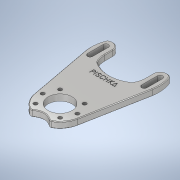
# Autodesk Inventor part: Motor Holder v3
Saved by Autodesk Inventor 2020.1 (Build 241239000, 239)
## iProperties
Created: 2019-03-01
Part Number: Motor Holder v3
Material: Aluminum 6061-AHC
Document SubType Name: Modeling
Designer: Petar
Density: 2.7 g/cm^3
Appearance: Aluminum - Dark
Mass: 26.5004 g
Surface Area: 70.5339 cm^2
Volume: 9.81495 cm^3
Author: Petar
Autodesk Inventor part; units mm, degrees
ref_plane "YZ Plane" through (0, 0, 0) normal (1, 0, 0) x (0, 1, 0)
ref_plane "XZ Plane" through (0, 0, 0) normal (0, 1, 0) x (-1, 0, 0)
ref_plane "XY Plane" through (0, 0, 0) normal (0, 0, 1) x (1, 0, 0)
sketch "Sketch1" plane through (0, 0, 0) normal (0, 1, 0) x (-1, 0, 0)
  line L0 (0, 0) -> (0, 51.5) construction
  circle A0 centre (0, 51.5) radius 9.5
  line L1 (16, -6.25) -> (16, 0)
  line L2 (21.5, 19.91967) -> (21.5, -14.08033) construction
  line L3 (-21.5, 18) -> (-21.5, -16) construction
  circle A1 centre (21.5, 3.5) radius 1.75 construction
  circle A2 centre (21.5, -3.5) radius 1.75 construction
  circle A3 centre (-21.5, 3.5) radius 1.75 construction
  circle A4 centre (-21.5, -3.5) radius 1.75 construction
  line L4 (-16, -6.25) -> (-16, 0)
  line L5 (21.5, 6.25) -> (21.5, -6.25) construction
  line L6 (19.45, 6.25) -> (19.45, -6.25)
  line L7 (23.55, -6.25) -> (23.55, 6.25)
  arc A5 (23.55, 6.25) -> (19.45, 6.25) centre (21.5, 6.25) ccw
  arc A6 (19.45, -6.25) -> (23.55, -6.25) centre (21.5, -6.25) ccw
  line L8 (-19.45, 6.25) -> (-19.45, -6.25)
  line L9 (-23.55, -6.25) -> (-23.55, 6.25)
  arc A7 (-19.45, 6.25) -> (-23.55, 6.25) centre (-21.5, 6.25) ccw
  arc A8 (-23.55, -6.25) -> (-19.45, -6.25) centre (-21.5, -6.25) ccw
  arc A9 (14.544724, 41.768556) -> (17.199681, 54.728155) centre (0, 51.5) ccw construction
  arc A10 (16, -6.25) -> (24.816002, -10.637953) centre (21.5, -6.25) ccw
  arc A11 (-24.816002, -10.637953) -> (-16, -6.25) centre (-21.5, -6.25) ccw
  line L10 (17.199681, 54.728155) -> (26.53665, 4.980583)
  line L11 (-17.199681, 54.728155) -> (-26.53665, 4.980583)
  circle A12 centre (0, 51.5) radius 13.75 construction
  circle A13 centre (9.722718, 61.222718) radius 1.5
  circle A14 centre (9.722718, 41.777282) radius 1.5
  line L12 (0, 51.5) -> (9.722718, 61.222718) construction
  line L13 (9.722718, 41.777282) -> (0, 51.5) construction
  circle A15 centre (-9.722718, 61.222718) radius 1.5
  circle A16 centre (-9.722718, 41.777282) radius 1.5
  circle A17 centre (13.75, 51.5) radius 1.5
  line L14 (13.75, 51.5) -> (0, 51.5) construction
  circle A18 centre (-13.75, 51.5) radius 1.5
  circle A19 centre (0, 22.942114) radius 1.5 construction
  line L15 (14.544724, 41.768556) -> (18.735106, 19.442114) construction
  arc A20 (17.199681, 54.728155) -> (-17.199681, 54.728155) centre (0, 51.5) ccw
  arc A21 (-17.199681, 54.728155) -> (-14.544724, 41.768556) centre (0, 51.5) ccw construction
  line L16 (-14.544724, 41.768556) -> (-18.735106, 19.442114) construction
  line L17 (7.5, 67.311388) -> (0, 61) construction
  line L18 (0, 61) -> (-7.5, 67.311388) construction
  spline S0 degree 2 poles (7.5, 67.311388) (0, 61) (-7.5, 67.311388) knots 1 1 1 2 2 2
  line L19 (7.5, 67.311388) -> (-7.5, 67.311388) construction
  line L20 (18.735106, 19.442114) -> (-18.735106, 19.442114) construction
  line L21 (18.735106, 19.442114) -> (11.806239, 33.884362) construction
  line L22 (14.544724, 41.768556) -> (12.108743, 38.127711) construction
  arc A22 (12.108743, 38.127711) -> (11.806239, 33.884362) centre (15.676028, 35.740946) ccw construction
  line L23 (-18.735106, 19.442114) -> (-11.806239, 33.884362) construction
  line L24 (-14.544724, 41.768556) -> (-12.108743, 38.127711) construction
  arc A23 (-11.806239, 33.884362) -> (-12.108743, 38.127711) centre (-15.676028, 35.740946) ccw construction
  line L25 (14.298579, 19.442114) -> (8.163141, 32.230571) construction
  line L26 (14.298579, 19.442114) -> (7.49461, 25.938983) construction
  line L27 (8.163141, 32.230571) -> (6.995239, 30.485011) construction
  arc A24 (6.995239, 30.485011) -> (7.49461, 25.938983) centre (9.94862, 28.508992) ccw construction
  line L28 (-14.298579, 19.442114) -> (-8.163141, 32.230571) construction
  line L29 (-14.298579, 19.442114) -> (-7.49461, 25.938983) construction
  line L30 (-8.163141, 32.230571) -> (-6.995239, 30.485011) construction
  arc A25 (-7.49461, 25.938983) -> (-6.995239, 30.485011) centre (-9.94862, 28.508992) ccw construction
  arc A26 (24.816002, -10.637953) -> (27, 0) centre (0, 0) ccw
  arc A27 (-24.816002, -10.637953) -> (24.816002, -10.637953) centre (0, 0) ccw construction
  arc A28 (-10.270866, 24.970168) -> (-26.53665, 4.980583) centre (0, 0) ccw construction
  line L31 (21.5, -11.75) -> (-21.5, -11.75) construction
  line L32 (-21.213203, 69) -> (25, 69) construction
  line L33 (0, 61) -> (0, 61) construction
  arc A29 (13.760985, 8.163043) -> (-13.760985, 8.163043) centre (0, -11.5) ccw
  line L34 (13.760985, 8.163043) -> (-13.760985, 8.163043) construction
  arc A30 (16, 0) -> (13.760985, 8.163043) centre (0, 0) ccw
  arc A31 (-13.760985, 8.163043) -> (-16, 0) centre (0, 0) ccw
  arc A32 (27, 0) -> (26.53665, 4.980583) centre (0, 0) ccw
  arc A33 (-27, 0) -> (-24.816002, -10.637953) centre (0, 0) ccw
  arc A34 (-26.53665, 4.980583) -> (-27, 0) centre (0, 0) ccw
  arc A35 (26.53665, 4.980583) -> (-12.029232, 24.172248) centre (0, 0) ccw construction
  line L35 (16, 0) -> (-16, 0) construction
  point P0 (21.5, 0)
  point P1 (0, 12.5)
  dimension "d1" = 19
  dimension "d0" = 51.5
  dimension "d3" = 3.5
  dimension "d4" = 3.5
  dimension "d5" = 7
  dimension "d9" = 3.5
  dimension "d11" = 32
  dimension "d15" = 4.1
  dimension "d24" = 3
  dimension "d25" = 3
  dimension "d27" = 45
  dimension "d29" = 3
  dimension "d30" = 3
  dimension "d50" = 15
  dimension "d53" = 27
  dimension "d75" = 80.75
  dimension "d76" = 8
  dimension "d78" = 0
  dimension "d81" = 6.25
  dimension "d82" = 12.5
  dimension "d85" = 5
  dimension "d86" = 4
  dimension "d98" = 15
  dimension "d99" = 24
  dimension "d101" = 43
  dimension "d104" = 2
  dimension "d105" = 27.5
  constraints: 70 end point, 58 point on circle, 35 centre point, 26 symmetric about line, 19 tangent, 13 point on line, 7 coincident, 5 horizontal, 5 vertical, 3 parallel, 2 perpendicular, 1 collinear, 1 midpoint, 1 vertical alignment, 16 other
  measures "d0" distance of L0.start L0.end
  measures "d3" diameter of A1
  measures "d4" diameter of A2
  measures "d5" distance of A2.centre A1.centre
  measures "d9" vertical distance of L0.start A1.centre
  measures "d11" distance between parallel lines of L4 L1
  measures "d15" distance between parallel lines of L6 L7
  measures "d24" diameter of A13
  measures "d25" diameter of A14
  measures "d27" angle of L0 L13
  measures "d29" diameter of A17
  measures "d30" diameter of A19
  measures "d50" distance of L17.start L18.end
  measures "d53" radius of A26
  measures "d75" distance between parallel lines of L31 L32
  measures "d78" distance of L33.start L33.end
  measures "d81" vertical distance of L5.start point (0, 12.5)
  measures "d82" distance of L5.end L5.start
  measures "d85" distance between parallel lines of L10 L15
  measures "d86" distance between parallel lines of L21 L25
  measures "d98" angle of L15 L21
  measures "d99" radius of A29
  measures "d101" distance of A4.centre A2.centre
  measures "d104" distance edge to line of A19 L20
  measures "d105" diameter of A12
extrude "Extrusion3" add sketch "Sketch1" along normal blind 5 contours L1 A30 A29 A31 L4 A11 A33 A34 L11 A20 S0 L10 A32 A26 A10
thread "Thread1" size "M3x0.5" class "6H" standard "ANSI Metric M Profile" full length
thread "Thread2" size "M3x0.5" class "6H" standard "ANSI Metric M Profile" full length
thread "Thread4" size "M3x0.5" class "6H" standard "ANSI Metric M Profile" full length
thread "Thread5" size "M3x0.5" class "6H" standard "ANSI Metric M Profile" full length
thread "Thread6" size "M3x0.5" class "6H" standard "ANSI Metric M Profile" full length
thread "Thread7" size "M3x0.5" class "6H" standard "ANSI Metric M Profile" full length
sketch "Sketch3" plane through (0, 5, 0) normal (0, 1, 0) x (1, 0, 0)
  line L0 (0, 0) -> (0, -51.5) construction
  circle A0 centre (0, -51.5) radius 9.5 construction
  arc A1 (-24.816002, 10.637953) -> (-26.53665, -4.980583) centre (0, 0) ccw construction
  line L1 (-7.003029, -18.212174) -> (-6.698457, -18.212174)
  line L2 (-7.003029, -14.734984) -> (-7.003029, -18.212174)
  line L3 (-6.698457, -18.212174) -> (-6.698457, -14.734984)
  spline S0 degree 3 poles (-5.654031, -15.648698) (-5.637534, -15.935503) (-5.515705, -16.141088) (-5.260627, -16.308603) knots 0 0 0 0 1 1 1 1
  spline S1 degree 3 poles (-5.04362, -16.066214) (-5.301236, -15.889817) (-5.388801, -15.600474) (-5.275855, -15.29971) knots 0 0 0 0 1 1 1 1
  spline S2 degree 3 poles (-5.275855, -15.29971) (-5.217479, -15.142348) (-5.041082, -15.007829) (-4.826613, -14.955798) knots 0 0 0 0 1 1 1 1
  spline S3 degree 3 poles (-4.858339, -14.684222) (-5.372303, -14.767979) (-5.68322, -15.143617) (-5.654031, -15.648698) knots 0 0 0 0 1 1 1 1
  spline S4 degree 3 poles (-4.744124, -14.665186) (-4.754277, -14.667724) (-4.806308, -14.676608) (-4.858339, -14.684222) knots 0 0 0 0 1 1 1 1
  line L4 (-6.698457, -14.734984) -> (-7.003029, -14.734984)
  line L5 (-9.769552, -16.702007) -> (-9.448483, -16.702007)
  spline S5 degree 3 poles (-9.448483, -16.702007) (-8.949748, -16.702007) (-8.673095, -16.669012) (-8.429438, -16.581448) knots 0 0 0 0 1 1 1 1
  line L6 (-10.074124, -14.732446) -> (-10.074124, -18.212174)
  line L7 (-9.769552, -18.212174) -> (-9.769552, -16.702007)
  line L8 (-10.074124, -18.212174) -> (-9.769552, -18.212174)
  spline S6 degree 3 poles (-7.845676, -15.941848) (-7.816488, -15.794638) (-7.826641, -15.519255) (-7.865981, -15.382198) knots 0 0 0 0 1 1 1 1
  spline S7 degree 3 poles (-8.429438, -16.581448) (-8.108369, -16.467233) (-7.906591, -16.246419) (-7.845676, -15.941848) knots 0 0 0 0 1 1 1 1
  spline S8 degree 3 poles (-7.865981, -15.382198) (-7.964967, -15.038286) (-8.199741, -14.854274) (-8.643907, -14.771786) knots 0 0 0 0 1 1 1 1
  spline S9 degree 3 poles (-8.161669, -15.648698) (-8.142633, -15.960884) (-8.256848, -16.186774) (-8.491621, -16.300988) knots 0 0 0 0 1 1 1 1
  spline S10 degree 3 poles (-8.623602, -15.062398) (-8.317762, -15.146155) (-8.183243, -15.318746) (-8.161669, -15.648698) knots 0 0 0 0 1 1 1 1
  spline S11 degree 3 poles (-8.491621, -16.300988) (-8.678171, -16.393629) (-8.81269, -16.410126) (-9.365995, -16.410126) knots 0 0 0 0 1 1 1 1
  line L9 (-9.365995, -16.410126) -> (-9.769552, -16.410126)
  line L10 (-9.769552, -16.410126) -> (-9.769552, -15.024327)
  spline S12 degree 3 poles (-4.528386, -16.300988) (-4.630505, -16.264595) (-4.739368, -16.222518) (-4.904133, -16.14744) (-4.983604, -16.107764) (-5.04362, -16.066214) knots -1.50825171 -1.50825171 -1.50825171 -1.50825171 -0.60874864 -0.60874864 0 0 0 0
  spline S13 degree 3 poles (-5.260627, -16.308603) (-5.126108, -16.397436) (-4.959863, -16.469772) (-4.598184, -16.595407) knots 0 0 0 0 1 1 1 1
  line L11 (-5.407836, -17.31115) -> (-5.735251, -17.31115)
  line L12 (-5.735251, -17.31115) -> (-5.726367, -17.370795)
  line L13 (-5.387532, -17.410136) -> (-5.407836, -17.31115)
  spline S14 degree 3 poles (-4.826613, -14.955798) (-4.706053, -14.925341) (-4.420517, -14.92661) (-4.280922, -14.955798) knots 0 0 0 0 1 1 1 1
  spline S15 degree 3 poles (-4.228891, -14.689298) (-4.321532, -14.671531) (-4.69717, -14.653765) (-4.744124, -14.665186) knots 0 0 0 0 1 1 1 1
  line L14 (-3.801222, -15.405041) -> (-3.785994, -15.483722)
  spline S16 degree 3 poles (-4.280922, -14.955798) (-4.010615, -15.014174) (-3.846908, -15.168998) (-3.801222, -15.405041) knots 0 0 0 0 1 1 1 1
  line L15 (-3.785994, -15.483722) -> (-3.473808, -15.483722)
  line L16 (-3.473808, -15.483722) -> (-3.482691, -15.435498)
  spline S17 degree 3 poles (-3.482691, -15.435498) (-3.523301, -15.198186) (-3.581677, -15.070012) (-3.708582, -14.943108) knots 0 0 0 0 1 1 1 1
  spline S18 degree 3 poles (-3.708582, -14.943108) (-3.845639, -14.807319) (-3.99031, -14.736253) (-4.228891, -14.689298) knots 0 0 0 0 1 1 1 1
  spline S19 degree 3 poles (-1.434449, -14.677877) (-1.881154, -14.750212) (-2.21872, -15.00656) (-2.428113, -15.430422) knots 0 0 0 0 1 1 1 1
  spline S20 degree 3 poles (-2.320244, -16.473579) (-2.320244, -15.682962) (-2.014404, -15.137272) (-1.487749, -14.986255) knots 0 0 0 0 1 1 1 1
  spline S21 degree 3 poles (-1.487749, -14.986255) (-1.402723, -14.962143) (-1.357037, -14.957067) (-1.190792, -14.957067) knots 0 0 0 0 1 1 1 1
  spline S22 degree 3 poles (-1.190792, -14.957067) (-1.01947, -14.957067) (-0.981399, -14.960874) (-0.898911, -14.986255) knots 0 0 0 0 1 1 1 1
  spline S23 degree 3 poles (-0.853225, -14.695643) (-0.991551, -14.661379) (-1.283432, -14.652496) (-1.434449, -14.677877) knots 0 0 0 0 1 1 1 1
  line L17 (-0.386216, -15.511641) -> (-0.378601, -15.547174)
  spline S24 degree 3 poles (-0.898911, -14.986255) (-0.612106, -15.077627) (-0.444592, -15.248948) (-0.386216, -15.511641) knots 0 0 0 0 1 1 1 1
  spline S25 degree 3 poles (-0.188244, -15.123312) (-0.32657, -14.91265) (-0.546116, -14.770517) (-0.853225, -14.695643) knots 0 0 0 0 1 1 1 1
  spline S26 degree 3 poles (-0.053725, -15.481184) (-0.068954, -15.370776) (-0.126061, -15.218491) (-0.188244, -15.123312) knots 0 0 0 0 1 1 1 1
  line L18 (-0.378601, -15.547174) -> (-0.044842, -15.547174)
  line L19 (-0.044842, -15.547174) -> (-0.053725, -15.481184)
  spline S27 degree 3 poles (-2.428113, -15.430422) (-2.64512, -15.869512) (-2.708572, -16.477386) (-2.594358, -17.033229) knots 0 0 0 0 1 1 1 1
  spline S28 degree 3 poles (-5.236515, -17.740088) (-5.299967, -17.661407) (-5.36342, -17.523081) (-5.387532, -17.410136) knots 0 0 0 0 1 1 1 1
  spline S29 degree 3 poles (-5.726367, -17.370795) (-5.699717, -17.553538) (-5.607077, -17.779428) (-5.505553, -17.905064) knots 0 0 0 0 1 1 1 1
  spline S30 degree 3 poles (-4.774582, -17.991359) (-4.867932, -17.973746) (-4.959865, -17.944336) (-5.117505, -17.858587) (-5.183697, -17.806111) (-5.236515, -17.740088) knots -1.49467749 -1.49467749 -1.49467749 -1.49467749 -0.70511356 -0.70511356 0 0 0 0
  spline S31 degree 3 poles (-5.505553, -17.905064) (-5.305043, -18.153797) (-4.956055, -18.288316) (-4.509351, -18.288316) knots 0 0 0 0 1 1 1 1
  spline S32 degree 3 poles (-9.245436, -15.029403) (-8.758121, -15.034479) (-8.716243, -15.037017) (-8.623602, -15.062398) knots 0 0 0 0 1 1 1 1
  spline S33 degree 3 poles (-8.643907, -14.771786) (-8.772081, -14.747674) (-8.846955, -14.743867) (-9.429447, -14.738791) knots 0 0 0 0 1 1 1 1
  line L20 (-9.429447, -14.738791) -> (-10.074124, -14.732446)
  line L21 (-9.769552, -15.024327) -> (-9.245436, -15.029403)
  spline S34 degree 3 poles (-0.731397, -17.893643) (-0.88622, -17.971055) (-0.975054, -17.99009) (-1.190792, -17.99009) knots 0 0 0 0 1 1 1 1
  spline S35 degree 3 poles (-0.386216, -17.434248) (-0.430632, -17.637295) (-0.558806, -17.806078) (-0.731397, -17.893643) knots 0 0 0 0 1 1 1 1
  spline S36 degree 3 poles (-1.108304, -18.28324) (-0.69967, -18.262936) (-0.36718, -18.09669) (-0.188244, -17.823845) knots 0 0 0 0 1 1 1 1
  line L22 (-0.378601, -17.399983) -> (-0.386216, -17.434248)
  line L23 (-0.046111, -17.399983) -> (-0.378601, -17.399983)
  line L24 (-0.054994, -17.465974) -> (-0.046111, -17.399983)
  spline S37 degree 3 poles (-0.188244, -17.823845) (-0.126061, -17.728667) (-0.070223, -17.57765) (-0.054994, -17.465974) knots 0 0 0 0 1 1 1 1
  line L25 (1.156946, -14.734984) -> (0.852375, -14.734984)
  line L26 (1.156946, -16.257841) -> (1.156946, -14.734984)
  line L27 (0.852375, -14.734984) -> (0.852375, -18.212174)
  line L28 (0.852375, -18.212174) -> (1.156946, -18.212174)
  line L29 (1.156946, -18.212174) -> (1.156946, -16.549722)
  line L30 (1.156946, -16.549722) -> (3.022446, -16.549722)
  line L31 (3.022446, -16.257841) -> (1.156946, -16.257841)
  line L32 (5.178557, -16.402512) -> (5.941255, -15.575093)
  line L33 (4.805457, -16.354288) -> (4.80165, -15.544636)
  spline S38 degree 3 poles (6.702683, -14.741329) (6.702683, -14.737522) (6.617657, -14.734984) (6.514864, -14.734984) knots 0 0 0 0 1 1 1 1
  spline S39 degree 3 poles (5.941255, -15.575093) (6.36004, -15.119505) (6.702683, -14.743867) (6.702683, -14.741329) knots 0 0 0 0 1 1 1 1
  line L34 (6.514864, -14.734984) -> (6.325776, -14.734984)
  line L35 (6.325776, -14.734984) -> (4.805457, -16.354288)
  line L36 (4.80165, -15.544636) -> (4.799112, -14.734984)
  line L37 (3.327017, -14.734984) -> (3.022446, -14.734984)
  line L38 (4.799112, -14.734984) -> (4.494541, -14.734984)
  line L39 (3.022446, -14.734984) -> (3.022446, -16.257841)
  line L40 (5.234395, -16.459619) -> (5.178557, -16.402512)
  spline S40 degree 3 poles (6.017397, -17.304805) (5.617648, -16.87206) (5.264852, -16.491345) (5.234395, -16.459619) knots 0 0 0 0 1 1 1 1
  line L41 (4.80165, -17.356836) -> (4.805457, -16.500229)
  line L42 (4.494541, -14.734984) -> (4.494541, -18.212174)
  line L43 (3.327017, -18.212174) -> (3.327017, -14.734984)
  line L44 (4.805457, -16.500229) -> (6.429838, -18.210905)
  line L45 (3.022446, -16.549722) -> (3.022446, -18.212174)
  line L46 (3.022446, -18.212174) -> (3.327017, -18.212174)
  line L47 (4.494541, -18.212174) -> (4.799112, -18.212174)
  line L48 (4.799112, -18.212174) -> (4.80165, -17.356836)
  line L49 (6.429838, -18.210905) -> (6.645576, -18.212174)
  spline S41 degree 3 poles (6.802938, -18.151259) (6.769943, -18.118264) (6.417147, -17.73755) (6.017397, -17.304805) knots 0 0 0 0 1 1 1 1
  line L50 (6.860045, -18.212174) -> (6.802938, -18.151259)
  line L51 (6.645576, -18.212174) -> (6.860045, -18.212174)
  spline S42 degree 3 poles (8.389247, -14.762903) (8.382902, -14.7794) (8.07833, -15.559865) (7.711576, -16.49896) knots 0 0 0 0 1 1 1 1
  spline S43 degree 3 poles (8.197621, -16.0053) (8.569452, -15.034479) (8.574528, -15.024327) (8.591026, -15.066205) knots 0 0 0 0 1 1 1 1
  spline S44 degree 3 poles (8.579604, -14.734984) (8.408283, -14.734984) (8.401938, -14.736253) (8.389247, -14.762903) knots 0 0 0 0 1 1 1 1
  line L52 (8.756002, -14.734984) -> (8.579604, -14.734984)
  line L53 (8.852449, -14.978641) -> (8.756002, -14.734984)
  spline S45 degree 3 poles (8.591026, -15.066205) (8.601178, -15.089048) (8.818185, -15.665195) (9.075802, -16.346674) knots 0 0 0 0 1 1 1 1
  spline S46 degree 3 poles (9.53139, -16.714698) (9.210321, -15.894893) (8.905749, -15.11316) (8.852449, -14.978641) knots 0 0 0 0 1 1 1 1
  spline S47 degree 3 poles (7.757261, -17.16521) (7.791526, -17.067493) (7.990766, -16.545914) (8.197621, -16.0053) knots 0 0 0 0 1 1 1 1
  line L54 (7.047864, -18.205828) -> (7.20015, -18.209636)
  spline S48 degree 3 poles (7.20015, -18.209636) (7.283907, -18.210905) (7.356242, -18.210905) (7.358781, -18.207097) knots 0 0 0 0 1 1 1 1
  line L55 (7.711576, -16.49896) -> (7.047864, -18.205828)
  spline S49 degree 3 poles (7.358781, -18.207097) (7.367664, -18.198214) (7.682388, -17.374602) (7.757261, -17.16521) knots 0 0 0 0 1 1 1 1
  spline S50 degree 3 poles (-4.193358, -17.9774) (-4.31011, -18.010395) (-4.632448, -18.018009) (-4.774582, -17.991359) knots 0 0 0 0 1 1 1 1
  ellipse E0 centre (-21.871561, 1.388012) end of major axis (-3.612492, -17.992801) minor radius 4.954361 (-4.509351, -18.288316) -> (-3.855791, -18.158874) ccw
  spline S51 degree 3 poles (-3.855791, -18.158874) (-3.769496, -18.116995) (-3.727618, -18.086538) (-3.645129, -18.00405) knots 0 0 0 0 1 1 1 1
  spline S52 degree 3 poles (-3.732694, -17.392369) (-3.752998, -17.708362) (-3.901477, -17.896181) (-4.193358, -17.9774) knots 0 0 0 0 1 1 1 1
  spline S53 degree 3 poles (-3.645129, -18.00405) (-3.478884, -17.837805) (-3.415432, -17.677905) (-3.402741, -17.392369) knots 0 0 0 0 1 1 1 1
  spline S54 degree 3 poles (-4.598184, -16.595407) (-4.264425, -16.710891) (-4.146403, -16.760383) (-4.028382, -16.833988) knots 0 0 0 0 1 1 1 1
  spline S55 degree 3 poles (-3.95097, -16.528148) (-4.062646, -16.47231) (-4.174322, -16.429162) (-4.528386, -16.300988) knots 0 0 0 0 1 1 1 1
  spline S56 degree 3 poles (-1.190792, -17.99009) (-1.357037, -17.99009) (-1.402723, -17.985014) (-1.487749, -17.960902) knots 0 0 0 0 1 1 1 1
  spline S57 degree 3 poles (-1.487749, -17.960902) (-2.014404, -17.809886) (-2.320244, -17.262926) (-2.320244, -16.473579) knots 0 0 0 0 1 1 1 1
  spline S58 degree 3 poles (-2.594358, -17.033229) (-2.423037, -17.863186) (-1.876077, -18.322581) (-1.108304, -18.28324) knots 0 0 0 0 1 1 1 1
  spline S59 degree 3 poles (-3.416701, -17.129676) (-3.475077, -16.868252) (-3.641322, -16.681702) (-3.95097, -16.528148) knots 0 0 0 0 1 1 1 1
  spline S60 degree 3 poles (-4.028382, -16.833988) (-3.807567, -16.971045) (-3.716196, -17.144905) (-3.732694, -17.392369) knots 0 0 0 0 1 1 1 1
  spline S61 degree 3 poles (-3.402741, -17.392369) (-3.397665, -17.261657) (-3.400203, -17.205819) (-3.416701, -17.129676) knots 0 0 0 0 1 1 1 1
  line L56 (8.203966, -17.920293) -> (8.153204, -18.063695)
  line L57 (8.153204, -18.063695) -> (8.103711, -18.205828)
  line L58 (8.103711, -18.205828) -> (8.601178, -18.209636)
  line L59 (8.936206, -17.917755) -> (8.203966, -17.920293)
  spline S62 degree 3 poles (9.075802, -16.346674) (9.333418, -17.026883) (9.571999, -17.6576) (9.606264, -17.748971) knots 0 0 0 0 1 1 1 1
  line L60 (9.669716, -17.913947) -> (8.936206, -17.917755)
  spline S63 degree 3 poles (8.601178, -18.209636) (8.875292, -18.210905) (9.327073, -18.210905) (9.606264, -18.209636) knots 0 0 0 0 1 1 1 1
  line L61 (9.606264, -17.748971) -> (9.669716, -17.913947)
  line L62 (9.606264, -18.209636) -> (10.113882, -18.205828)
  line L63 (10.113882, -18.205828) -> (9.53139, -16.714698)
  point P0 (0, -22.942114)
  constraints: 128 end point, 2 coincident, 2 horizontal alignment, 1 vertical, 194 other
emboss "Emboss1" sketch "Sketch3" operation cut depth 0.5 direction (0, -1, 0)
sketch "Sketch4" plane through (0, 0, 0) normal (0, -1, 0) x (1, 0, 0)
  circle A0 centre (0, 51.5) radius 9.5 construction
  arc A1 (24.816002, -10.637953) -> (26.53665, 4.980583) centre (0, 0) ccw construction
  line L0 (0, 0) -> (0, 51.5) construction
  spline S0 degree 3 poles (8.012999, 15.717163) (7.983811, 15.569954) (7.993964, 15.294571) (8.033304, 15.157513) knots 0 0 0 0 1 1 1 1
  spline S1 degree 3 poles (8.596761, 16.356763) (8.275692, 16.242549) (8.073914, 16.021735) (8.012999, 15.717163) knots 0 0 0 0 1 1 1 1
  spline S2 degree 3 poles (8.328992, 15.424013) (8.309956, 15.736199) (8.424171, 15.962089) (8.658945, 16.076304) knots 0 0 0 0 1 1 1 1
  spline S3 degree 3 poles (8.790925, 14.837713) (8.485085, 14.921471) (8.350566, 15.094061) (8.328992, 15.424013) knots 0 0 0 0 1 1 1 1
  spline S4 degree 3 poles (8.033304, 15.157513) (8.13229, 14.813602) (8.367064, 14.62959) (8.81123, 14.547102) knots 0 0 0 0 1 1 1 1
  spline S5 degree 3 poles (9.615806, 16.477323) (9.117071, 16.477323) (8.840418, 16.444328) (8.596761, 16.356763) knots 0 0 0 0 1 1 1 1
  line L1 (9.936875, 16.477323) -> (9.615806, 16.477323)
  line L2 (9.936875, 17.987489) -> (9.936875, 16.477323)
  line L3 (10.241447, 17.987489) -> (9.936875, 17.987489)
  line L4 (10.241447, 14.507761) -> (10.241447, 17.987489)
  spline S6 degree 3 poles (8.658945, 16.076304) (8.845494, 16.168944) (8.980014, 16.185442) (9.533318, 16.185442) knots 0 0 0 0 1 1 1 1
  line L5 (9.533318, 16.185442) -> (9.936875, 16.185442)
  spline S7 degree 3 poles (9.412759, 14.804718) (8.925444, 14.809794) (8.883566, 14.812333) (8.790925, 14.837713) knots 0 0 0 0 1 1 1 1
  line L6 (9.936875, 16.185442) -> (9.936875, 14.799642)
  spline S8 degree 3 poles (8.81123, 14.547102) (8.939404, 14.52299) (9.014278, 14.519183) (9.596771, 14.514106) knots 0 0 0 0 1 1 1 1
  line L7 (9.936875, 14.799642) -> (9.412759, 14.804718)
  line L8 (9.596771, 14.514106) -> (10.241447, 14.507761)
  spline S9 degree 3 poles (4.911448, 14.440502) (4.9216, 14.44304) (4.973631, 14.451923) (5.025662, 14.459537) knots 0 0 0 0 1 1 1 1
  spline S10 degree 3 poles (4.993936, 14.731114) (4.873376, 14.700656) (4.58784, 14.701925) (4.448245, 14.731114) knots 0 0 0 0 1 1 1 1
  spline S11 degree 3 poles (3.875905, 14.718423) (4.012962, 14.582635) (4.157633, 14.511568) (4.396214, 14.464614) knots 0 0 0 0 1 1 1 1
  spline S12 degree 3 poles (4.396214, 14.464614) (4.488855, 14.446847) (4.864493, 14.42908) (4.911448, 14.440502) knots 0 0 0 0 1 1 1 1
  spline S13 degree 3 poles (4.448245, 14.731114) (4.177938, 14.78949) (4.014231, 14.944313) (3.968545, 15.180356) knots 0 0 0 0 1 1 1 1
  line L9 (3.968545, 15.180356) -> (3.953317, 15.259037)
  spline S14 degree 3 poles (4.118293, 16.303463) (4.229969, 16.247625) (4.341645, 16.204478) (4.695709, 16.076304) knots 0 0 0 0 1 1 1 1
  spline S15 degree 3 poles (4.765507, 16.370723) (4.431748, 16.486206) (4.313726, 16.535699) (4.195705, 16.609304) knots 0 0 0 0 1 1 1 1
  line L10 (3.953317, 15.259037) -> (3.641131, 15.259037)
  line L11 (3.641131, 15.259037) -> (3.650014, 15.210813)
  spline S16 degree 3 poles (3.584024, 16.904992) (3.6424, 16.643568) (3.808645, 16.457018) (4.118293, 16.303463) knots 0 0 0 0 1 1 1 1
  spline S17 degree 3 poles (4.195705, 16.609304) (3.974891, 16.746361) (3.883519, 16.92022) (3.900017, 17.167685) knots 0 0 0 0 1 1 1 1
  spline S18 degree 3 poles (3.570064, 17.167685) (3.564988, 17.036973) (3.567526, 16.981135) (3.584024, 16.904992) knots 0 0 0 0 1 1 1 1
  spline S19 degree 3 poles (1.601772, 14.453192) (2.048477, 14.525528) (2.386043, 14.781875) (2.595436, 15.205737) knots 0 0 0 0 1 1 1 1
  spline S20 degree 3 poles (2.595436, 15.205737) (2.812443, 15.644828) (2.875896, 16.252701) (2.761681, 16.808544) knots 0 0 0 0 1 1 1 1
  spline S21 degree 3 poles (2.487567, 16.248894) (2.487567, 15.458278) (2.181727, 14.912587) (1.655072, 14.761571) knots 0 0 0 0 1 1 1 1
  spline S22 degree 3 poles (3.812453, 17.779365) (3.646207, 17.61312) (3.582755, 17.45322) (3.570064, 17.167685) knots 0 0 0 0 1 1 1 1
  spline S23 degree 3 poles (1.655072, 17.736218) (2.181727, 17.585201) (2.487567, 17.038242) (2.487567, 16.248894) knots 0 0 0 0 1 1 1 1
  spline S24 degree 3 poles (1.358115, 17.765406) (1.52436, 17.765406) (1.570046, 17.76033) (1.655072, 17.736218) knots 0 0 0 0 1 1 1 1
  spline S25 degree 3 poles (2.761681, 16.808544) (2.59036, 17.638501) (2.0434, 18.097896) (1.275627, 18.058556) knots 0 0 0 0 1 1 1 1
  spline S26 degree 3 poles (3.650014, 15.210813) (3.690624, 14.973502) (3.749, 14.845328) (3.875905, 14.718423) knots 0 0 0 0 1 1 1 1
  line L12 (0.545924, 15.32249) -> (0.212165, 15.32249)
  line L13 (0.553539, 15.286956) -> (0.545924, 15.32249)
  line L14 (0.212165, 15.32249) -> (0.221048, 15.256499)
  spline S27 degree 3 poles (0.221048, 15.256499) (0.236277, 15.146092) (0.293384, 14.993806) (0.355567, 14.898628) knots 0 0 0 0 1 1 1 1
  spline S28 degree 3 poles (1.066234, 14.761571) (0.779429, 14.852942) (0.611915, 15.024263) (0.553539, 15.286956) knots 0 0 0 0 1 1 1 1
  spline S29 degree 3 poles (0.355567, 14.898628) (0.493894, 14.687966) (0.713439, 14.545833) (1.020548, 14.470959) knots 0 0 0 0 1 1 1 1
  line L15 (-0.989623, 16.033156) -> (-0.989623, 14.510299)
  line L16 (-0.989623, 14.510299) -> (-0.685051, 14.510299)
  spline S30 degree 3 poles (1.655072, 14.761571) (1.570046, 14.737459) (1.52436, 14.732383) (1.358115, 14.732383) knots 0 0 0 0 1 1 1 1
  spline S31 degree 3 poles (1.358115, 14.732383) (1.186793, 14.732383) (1.148722, 14.73619) (1.066234, 14.761571) knots 0 0 0 0 1 1 1 1
  spline S32 degree 3 poles (1.020548, 14.470959) (1.158874, 14.436695) (1.450755, 14.427811) (1.601772, 14.453192) knots 0 0 0 0 1 1 1 1
  line L17 (-0.685051, 14.510299) -> (-0.685051, 17.987489)
  line L18 (0.213434, 17.175299) -> (0.545924, 17.175299)
  line L19 (0.545924, 17.175299) -> (0.553539, 17.209563)
  line L20 (0.222317, 17.241289) -> (0.213434, 17.175299)
  line L21 (-0.989623, 17.987489) -> (-0.989623, 16.325037)
  line L22 (-0.685051, 17.987489) -> (-0.989623, 17.987489)
  spline S33 degree 3 poles (0.553539, 17.209563) (0.597955, 17.412611) (0.726129, 17.581394) (0.89872, 17.668958) knots 0 0 0 0 1 1 1 1
  spline S34 degree 3 poles (0.89872, 17.668958) (1.053543, 17.74637) (1.142377, 17.765406) (1.358115, 17.765406) knots 0 0 0 0 1 1 1 1
  spline S35 degree 3 poles (1.275627, 18.058556) (0.866993, 18.038251) (0.534503, 17.872006) (0.355567, 17.599161) knots 0 0 0 0 1 1 1 1
  spline S36 degree 3 poles (0.355567, 17.599161) (0.293384, 17.503982) (0.237546, 17.352965) (0.222317, 17.241289) knots 0 0 0 0 1 1 1 1
  line L23 (7.170352, 17.987489) -> (6.865781, 17.987489)
  line L24 (7.170352, 14.510299) -> (7.170352, 17.987489)
  line L25 (6.865781, 17.987489) -> (6.865781, 14.510299)
  spline S37 degree 3 poles (5.821355, 15.424013) (5.804857, 15.710818) (5.683028, 15.916404) (5.42795, 16.083918) knots 0 0 0 0 1 1 1 1
  spline S38 degree 3 poles (5.210943, 15.84153) (5.468559, 15.665132) (5.556124, 15.37579) (5.443178, 15.075025) knots 0 0 0 0 1 1 1 1
  line L26 (6.865781, 14.510299) -> (7.170352, 14.510299)
  line L27 (5.902574, 17.086465) -> (5.89369, 17.146111)
  spline S39 degree 3 poles (5.89369, 17.146111) (5.86704, 17.328854) (5.7744, 17.554744) (5.672876, 17.68038) knots 0 0 0 0 1 1 1 1
  line L28 (5.575159, 17.086465) -> (5.902574, 17.086465)
  spline S40 degree 3 poles (5.025662, 14.459537) (5.539626, 14.543294) (5.850543, 14.918933) (5.821355, 15.424013) knots 0 0 0 0 1 1 1 1
  spline S41 degree 3 poles (5.443178, 15.075025) (5.384802, 14.917663) (5.208405, 14.783144) (4.993936, 14.731114) knots 0 0 0 0 1 1 1 1
  line L29 (5.554855, 17.185451) -> (5.575159, 17.086465)
  spline S42 degree 3 poles (5.403838, 17.515404) (5.46729, 17.436723) (5.530743, 17.298396) (5.554855, 17.185451) knots 0 0 0 0 1 1 1 1
  line L30 (-0.989623, 16.325037) -> (-2.855123, 16.325037)
  line L31 (-2.855123, 16.033156) -> (-0.989623, 16.033156)
  line L32 (-4.638134, 16.129604) -> (-4.634327, 15.319952)
  line L33 (-4.631789, 14.510299) -> (-4.327218, 14.510299)
  line L34 (-4.634327, 15.319952) -> (-4.631789, 14.510299)
  line L35 (-5.011234, 16.177828) -> (-5.773932, 15.350409)
  line L36 (-6.158453, 14.510299) -> (-4.638134, 16.129604)
  line L37 (-6.347541, 14.510299) -> (-6.158453, 14.510299)
  spline S43 degree 3 poles (-6.53536, 14.516645) (-6.53536, 14.512837) (-6.450334, 14.510299) (-6.347541, 14.510299) knots 0 0 0 0 1 1 1 1
  spline S44 degree 3 poles (-5.773932, 15.350409) (-6.192717, 14.894821) (-6.53536, 14.519183) (-6.53536, 14.516645) knots 0 0 0 0 1 1 1 1
  line L38 (-2.855123, 17.987489) -> (-3.159694, 17.987489)
  line L39 (-2.855123, 16.325037) -> (-2.855123, 17.987489)
  line L40 (-2.855123, 14.510299) -> (-2.855123, 16.033156)
  line L41 (-3.159694, 14.510299) -> (-2.855123, 14.510299)
  line L42 (-3.159694, 17.987489) -> (-3.159694, 14.510299)
  line L43 (-4.327218, 14.510299) -> (-4.327218, 17.987489)
  line L44 (-4.327218, 17.987489) -> (-4.631789, 17.987489)
  line L45 (-4.631789, 17.987489) -> (-4.634327, 17.132151)
  line L46 (-4.634327, 17.132151) -> (-4.638134, 16.275544)
  line L47 (-6.880541, 17.981144) -> (-7.032827, 17.984951)
  spline S45 degree 3 poles (-7.032827, 17.984951) (-7.116584, 17.98622) (-7.188919, 17.98622) (-7.191458, 17.982413) knots 0 0 0 0 1 1 1 1
  spline S46 degree 3 poles (-7.191458, 17.982413) (-7.200341, 17.97353) (-7.515065, 17.149918) (-7.589938, 16.940525) knots 0 0 0 0 1 1 1 1
  spline S47 degree 3 poles (-7.589938, 16.940525) (-7.624203, 16.842808) (-7.823443, 16.32123) (-8.030298, 15.780616) knots 0 0 0 0 1 1 1 1
  line L48 (-7.985881, 17.839011) -> (-7.936388, 17.981144)
  line L49 (-8.036643, 17.695608) -> (-7.985881, 17.839011)
  line L50 (-7.544253, 16.274275) -> (-6.880541, 17.981144)
  spline S48 degree 3 poles (-8.221924, 14.538218) (-8.215579, 14.554716) (-7.911007, 15.33518) (-7.544253, 16.274275) knots 0 0 0 0 1 1 1 1
  spline S49 degree 3 poles (-8.030298, 15.780616) (-8.402129, 14.809794) (-8.407205, 14.799642) (-8.423703, 14.841521) knots 0 0 0 0 1 1 1 1
  spline S50 degree 3 poles (-8.412281, 14.510299) (-8.24096, 14.510299) (-8.234614, 14.511568) (-8.221924, 14.538218) knots 0 0 0 0 1 1 1 1
  line L51 (-7.936388, 17.981144) -> (-8.433855, 17.984951)
  line L52 (-8.768883, 17.69307) -> (-8.036643, 17.695608)
  line L53 (-8.588679, 14.510299) -> (-8.412281, 14.510299)
  line L54 (-8.685126, 14.753956) -> (-8.588679, 14.510299)
  spline S51 degree 3 poles (-8.423703, 14.841521) (-8.433855, 14.864363) (-8.650862, 15.440511) (-8.908479, 16.121989) knots 0 0 0 0 1 1 1 1
  spline S52 degree 3 poles (-9.364067, 16.490013) (-9.042998, 15.670209) (-8.738426, 14.888475) (-8.685126, 14.753956) knots 0 0 0 0 1 1 1 1
  spline S53 degree 3 poles (-8.908479, 16.121989) (-9.166095, 16.802199) (-9.404676, 17.432915) (-9.43894, 17.524287) knots 0 0 0 0 1 1 1 1
  spline S54 degree 3 poles (-8.433855, 17.984951) (-8.707969, 17.98622) (-9.15975, 17.98622) (-9.43894, 17.984951) knots 0 0 0 0 1 1 1 1
  line L55 (-9.502393, 17.689263) -> (-8.768883, 17.69307)
  line L56 (-9.43894, 17.524287) -> (-9.502393, 17.689263)
  line L57 (-9.946559, 17.981144) -> (-9.364067, 16.490013)
  line L58 (-9.43894, 17.984951) -> (-9.946559, 17.981144)
  line L59 (-5.067072, 16.234935) -> (-5.011234, 16.177828)
  spline S55 degree 3 poles (-5.850074, 17.08012) (-5.450324, 16.647375) (-5.097529, 16.266661) (-5.067072, 16.234935) knots 0 0 0 0 1 1 1 1
  line L60 (-4.638134, 16.275544) -> (-6.262515, 17.98622)
  spline S56 degree 3 poles (-6.635615, 17.926575) (-6.60262, 17.89358) (-6.249824, 17.512865) (-5.850074, 17.08012) knots 0 0 0 0 1 1 1 1
  line L61 (-6.262515, 17.98622) -> (-6.478253, 17.987489)
  line L62 (-6.692722, 17.987489) -> (-6.635615, 17.926575)
  line L63 (-6.478253, 17.987489) -> (-6.692722, 17.987489)
  spline S57 degree 3 poles (4.695709, 16.076304) (4.797828, 16.03991) (4.906692, 15.997834) (5.071456, 15.922756) (5.150927, 15.883079) (5.210943, 15.84153) knots -1.50825171 -1.50825171 -1.50825171 -1.50825171 -0.60874864 -0.60874864 0 0 0 0
  spline S58 degree 3 poles (5.42795, 16.083918) (5.293431, 16.172751) (5.127186, 16.245087) (4.765507, 16.370723) knots 0 0 0 0 1 1 1 1
  spline S59 degree 3 poles (4.023114, 17.934189) (3.936819, 17.892311) (3.894941, 17.861853) (3.812453, 17.779365) knots 0 0 0 0 1 1 1 1
  spline S60 degree 3 poles (4.360681, 17.752715) (4.477433, 17.785711) (4.799771, 17.793325) (4.941905, 17.766675) knots 0 0 0 0 1 1 1 1
  ellipse E0 centre (22.038884, -1.612697) end of major axis (3.779815, 17.768117) minor radius 4.954361 (4.676674, 18.063632) -> (4.023114, 17.934189) ccw
  spline S61 degree 3 poles (4.941905, 17.766675) (5.035255, 17.749062) (5.127188, 17.719652) (5.284828, 17.633903) (5.35102, 17.581426) (5.403838, 17.515404) knots -1.49467749 -1.49467749 -1.49467749 -1.49467749 -0.70511356 -0.70511356 0 0 0 0
  spline S62 degree 3 poles (5.672876, 17.68038) (5.472366, 17.929113) (5.123378, 18.063632) (4.676674, 18.063632) knots 0 0 0 0 1 1 1 1
  spline S63 degree 3 poles (3.900017, 17.167685) (3.920322, 17.483677) (4.0688, 17.671496) (4.360681, 17.752715) knots 0 0 0 0 1 1 1 1
  constraints: 128 end point, 2 horizontal alignment, 1 vertical, 194 other
emboss "Emboss2" sketch "Sketch4" operation cut depth 0.5 direction (0, 1, 0)
fillet "Fillet3" [suppressed]
fillet "Fillet5" radius 2 6 edges at (-7.5, 2.5, 67.3114) (7.5, 2.5, 67.3114) (24.816, 2.5, -10.638) (-24.816, 2.5, -10.638) (-13.761, 2.5, 8.163) (13.761, 2.5, 8.163)
chamfer "Chamfer3" distance 0.5 angle 45 40 edges at (14.2685, 5, 61.6321) (21.8682, 5, 29.8544) (26.8705, 5, -2.6415) (24.7034, 5, -10.6299) (18.713, 5, -10.9916) (16, 5, -3.125) (15.4929, 5, 3.9962) (13.7269, 5, 8.124) (0, 5, 12.5) (7.6088, 5, 66.9375) (0, 5, 64.1557) (-7.6088, 5, 66.9375) (-14.2685, 5, 61.6321) (-21.8682, 5, 29.8544) (-26.8705, 5, -2.6415) (-24.7034, 5, -10.6299) (-18.713, 5, -10.9916) (-16, 5, -3.125) (-15.4929, 5, 3.9962) (-13.7269, 5, 8.124) (0, 0, 64.1557) (7.6088, 0, 66.9375) (14.2685, 0, 61.6321) (21.8682, 0, 29.8544) (26.8705, 0, -2.6415) (24.7034, 0, -10.6299) (18.713, 0, -10.9916) (16, 0, -3.125) (15.4929, 0, 3.9962) (13.7269, 0, 8.124) (0, 0, 12.5) (-7.6088, 0, 66.9375) (-14.2685, 0, 61.6321) (-21.8682, 0, 29.8544) (-26.8705, 0, -2.6415) (-24.7034, 0, -10.6299) (-18.713, 0, -10.9916) (-16, 0, -3.125) (-15.4929, 0, 3.9962) (-13.7269, 0, 8.124)
sketch "Center Lines" plane through (0, 5, 0) normal (0, 1, 0) x (1, 0, 0)
  arc A0 (-23.55, -6.25) -> (-19.45, -6.25) centre (-21.5, -6.25) ccw construction
  line L0 (-23.55, -6.25) -> (-23.55, 6.25) construction
  arc A1 (-19.45, 6.25) -> (-23.55, 6.25) centre (-21.5, 6.25) ccw construction
  line L1 (-19.45, 6.25) -> (-19.45, -6.25) construction
  line L2 (-21.5, -6.25) -> (-21.5, 6.25) construction
  line L3 (19.45, -6.25) -> (19.45, 6.25) construction
  arc A2 (19.45, -6.25) -> (23.55, -6.25) centre (21.5, -6.25) ccw construction
  line L4 (23.55, 6.25) -> (23.55, -6.25) construction
  arc A3 (23.55, 6.25) -> (19.45, 6.25) centre (21.5, 6.25) ccw construction
  line L5 (21.5, -6.25) -> (21.5, 6.25) construction
  constraints: 4 end point, 2 vertical
body "Solid3"
